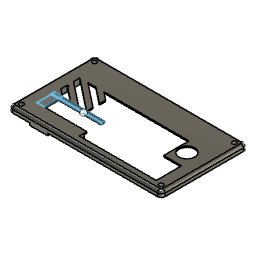
Untitled v9 (Autodesk Fusion 360 archive; units mm, degrees)
design "top"
Autodesk Fusion 360 part; units mm, degrees
sketch "Sketch1" plane through (0, 0, 0) normal (0, 0, 1) x (1, 0, 0)
  line L0 (0, 0) -> (119.41, 0)
  line L1 (119.41, 0) -> (119.41, 67.24)
  line L2 (119.41, 67.24) -> (0, 67.24)
  line L3 (0, 67.24) -> (0, 0)
  line L4 (0, 0) -> (5, 0)
  line L5 (5, 0) -> (5, 5)
  line L6 (5, 5) -> (0, 5)
  line L7 (0, 5) -> (0, 0)
  circle A0 centre (5, 5) radius 1.7
  line L8 (0, 67.24) -> (5, 67.24)
  line L9 (5, 67.24) -> (5, 62.24)
  line L10 (5, 62.24) -> (0, 62.24)
  line L11 (0, 62.24) -> (0, 67.24)
  circle A1 centre (5, 62.24) radius 1.7
  line L12 (119.41, 67.24) -> (114.41, 67.24)
  line L13 (114.41, 67.24) -> (114.41, 62.24)
  line L14 (114.41, 62.24) -> (119.41, 62.24)
  line L15 (119.41, 62.24) -> (119.41, 67.24)
  circle A2 centre (114.41, 62.24) radius 1.7
  line L16 (119.41, 0) -> (114.41, 0)
  line L17 (114.41, 0) -> (114.41, 5)
  line L18 (114.41, 5) -> (119.41, 5)
  line L19 (119.41, 5) -> (119.41, 0)
  circle A3 centre (114.41, 5) radius 1.7
  line L20 (0, 62.24) -> (10, 62.24)
  line L21 (0, 67.24) -> (10, 67.24)
  line L22 (10, 67.24) -> (10, 57.24)
  line L23 (10, 57.24) -> (0, 57.24)
  line L24 (0, 57.24) -> (0, 67.24)
  line L25 (0, 0) -> (10, 0)
  line L26 (10, 0) -> (10, 10)
  line L27 (10, 10) -> (0, 10)
  line L28 (0, 10) -> (0, 0)
  line L29 (119.41, 0) -> (109.41, 0)
  line L30 (109.41, 0) -> (109.41, 10)
  line L31 (109.41, 10) -> (119.41, 10)
  line L32 (119.41, 10) -> (119.41, 0)
  line L33 (10, 57.24) -> (109.41, 57.24)
  line L34 (109.41, 57.24) -> (109.41, 10)
  line L35 (109.41, 10) -> (10, 10)
  line L36 (10, 10) -> (10, 57.24)
  line L37 (109.41, 10) -> (109.41, 6.042)
  line L38 (109.41, 6.042) -> (49.127, 6.042)
  line L39 (49.127, 6.042) -> (49.127, 25.842)
  line L40 (49.127, 25.842) -> (109.41, 25.842)
  line L41 (109.41, 25.842) -> (109.41, 6.042)
  line L42 (109.41, 25.842) -> (95.41, 25.842)
  line L43 (95.41, 25.842) -> (35.127, 25.842)
  line L44 (35.127, 25.842) -> (35.127, 45.642)
  line L45 (35.127, 45.642) -> (95.41, 45.642)
  line L46 (95.41, 45.642) -> (95.41, 25.842)
  line L47 (35.127, 45.642) -> (10, 45.642)
  line L48 (10, 10) -> (49.127, 10)
  line L49 (49.127, 10) -> (49.127, 12)
  line L50 (49.127, 12) -> (10, 12)
  line L51 (10, 12) -> (10, 10)
  line L52 (10, 45.642) -> (11.5, 45.642)
  line L53 (11.5, 45.642) -> (11.5, 12)
  line L54 (11.5, 12) -> (10, 12)
  line L55 (10, 12) -> (10, 45.642)
  line L56 (35.127, 25.842) -> (10, 25.842)
  line L57 (22.5635, 45.642) -> (35.127, 35.742)
  line L58 (22.5635, 45.642) -> (10, 45.642)
  line L59 (35.127, 35.742) -> (35.127, 25.842)
  line L60 (16.2818, 45.642) -> (35.127, 30.792)
  line L61 (22.5635, 45.642) -> (35.127, 45.642)
  line L62 (28.8453, 45.642) -> (35.127, 40.692)
  line L63 (10, 45.642) -> (35.127, 25.842)
  line L64 (10, 45.642) -> (10, 25.842)
  line L65 (10, 45.642) -> (10, 33.62)
  line L66 (35.127, 35.742) -> (10, 35.742)
  line L67 (10, 45.642) -> (10, 35.742)
  line L68 (22.5635, 25.842) -> (35.127, 25.842)
  line L69 (28.8453, 25.842) -> (10, 40.692)
  line L70 (22.5635, 25.842) -> (10, 35.742)
  line L71 (10, 25.842) -> (22.5635, 25.842)
  line L72 (10, 35.742) -> (10, 25.842)
  line L73 (10, 30.792) -> (16.2817, 25.842)
  dimension "d1" = 119.41
  dimension "d2" = 67.24
  dimension "d3" = 5
  dimension "d4" = 5
  dimension "d5" = 3.4
  dimension "d6" = 5
  dimension "d7" = 5
  dimension "d8" = 3.4
  dimension "d9" = 5
  dimension "d10" = 5
  dimension "d11" = 3.4
  dimension "d12" = 5
  dimension "d13" = 5
  dimension "d14" = 3.4
  dimension "d15" = 10
  dimension "d16" = 10
  dimension "d17" = 10
  dimension "d18" = 10
  dimension "d19" = 10
  dimension "d20" = 10
  dimension "d21" = 3.958
  dimension "d22" = 60.283
  dimension "d23" = 19.8
  dimension "d24" = 14
  dimension "d25" = 60.283
  dimension "d26" = 19.8
  dimension "d27" = 2
  dimension "d28" = 1.5
  dimension "d29" = 90
  constraint horizontal L0
  constraint vertical L1
  constraint horizontal L2
  constraint vertical L3
  constraint coincident L0.start L3.end
  constraint horizontal L4
  constraint vertical L5
  constraint horizontal L6
  constraint vertical L7
  constraint coincident L5.end L6.start
  constraint horizontal L8
  constraint vertical L9
  constraint horizontal L10
  constraint vertical L11
  constraint coincident L9.end L10.start
  constraint horizontal L12
  constraint vertical L13
  constraint horizontal L14
  constraint vertical L15
  constraint coincident L13.end L14.start
  constraint horizontal L16
  constraint vertical L17
  constraint horizontal L18
  constraint vertical L19
  constraint coincident L17.end L18.start
  constraint perpendicular L11 L20
  constraint horizontal L21
  constraint vertical L22
  constraint horizontal L23
  constraint vertical L24
  constraint horizontal L25
  constraint vertical L26
  constraint horizontal L27
  constraint vertical L28
  constraint horizontal L29
  constraint vertical L30
  constraint horizontal L31
  constraint vertical L32
  constraint horizontal L33
  constraint vertical L34
  constraint horizontal L35
  constraint vertical L36
  constraint perpendicular L31 L37
  constraint horizontal L38
  constraint vertical L39
  constraint horizontal L40
  constraint vertical L41
  constraint perpendicular L41 L42
  constraint horizontal L43
  constraint vertical L44
  constraint horizontal L45
  constraint vertical L46
  constraint coincident L36 L47.end
  constraint perpendicular L36 L47
  constraint horizontal L48
  constraint vertical L49
  constraint horizontal L50
  constraint vertical L51
  constraint horizontal L52
  constraint vertical L53
  constraint horizontal L54
  constraint vertical L55
  constraint coincident L50 L53.end
  constraint coincident L36 L56.end
  constraint perpendicular L36 L56
  constraint midpoint L47 L57.start
  constraint midpoint L44 L57.end
  constraint midpoint L58 L60.start
  constraint midpoint L59 L60.end
  constraint midpoint L61 L62.start
  constraint coincident L44 L62.end
  constraint parallel L60 L62
  constraint midpoint L36 L65.end
  constraint coincident L65 L66.end
  constraint midpoint L56 L68.start
  constraint midpoint L68 L69.start
  constraint midpoint L67 L69.end
  constraint midpoint L72 L73.start
  constraint midpoint L71 L73.end
  measures "d1" distance of L0.start L0.end
  measures "d2" distance of L0.start L2.end
  measures "d3" distance of L0.start L4.end
  measures "d4" distance of L0.start L6.end
  measures "d5" diameter of A0
  measures "d6" distance of L2.end L8.end
  measures "d7" distance of L2.end L10.end
  measures "d8" diameter of A1
  measures "d9" distance of L1.end L12.end
  measures "d10" distance of L1.end L14.end
  measures "d11" diameter of A2
  measures "d12" distance of L0.end L16.end
  measures "d13" distance of L0.end L18.end
  measures "d14" diameter of A3
  measures "d15" distance of L2.end L21.end
  measures "d16" distance of L2.end L23.end
  measures "d17" distance of L0.start L25.end
  measures "d18" distance of L0.start L27.end
  measures "d19" distance of L0.end L29.end
  measures "d20" distance of L0.end L31.end
  measures "d21" distance of L30.end L37.end
  measures "d22" distance of L37.end L38.end
  measures "d23" distance of L37.end L40.end
  measures "d24" distance of L40.end L42.end
  measures "d25" distance of L42.end L43.end
  measures "d26" distance of L42.end L45.end
  measures "d27" distance of L26.end L50.end
  measures "d28" distance of L47.end L52.end
  measures "d29" angle of L65 L66
extrude "Extrude1" add sketch "Sketch1" against normal blind 4.5 contours L0 L3 L4 L5 L6 L7 A0 L25 L28 | L0 L3 L5 L6 A0 L25 L26 L27 L28 | L0 L26 L30 L35 L38 L39 L48 | L3 L23 L27 L36 L51 L55 L64 L65 L67 L72 | L0 L1 L17 L18 A3 L29 L30 L31 L32 L37 L41 | L3 L10 A1 L20 L22 L23 L24 | L0 L1 L16 L17 L18 L19 A3 L29 L32 | L2 L3 L8 L9 L10 L11 A1 L20 L21 L24 | L1 L2 L13 L14 A2 L22 L31 L33 L34 L41 | L2 L9 A1 L20 L21 L22 | L1 L2 L12 L13 L14 L15 A2
extrude "Extrude2" add sketch "Sketch1" against normal blind 1 contours L35 L36 L39 L48 L49 L50 L51 L54 | L33 L34 L36 L40 L42 L45 L46 L47 L52 L58 L61 | L36 L53 L55 L56 L64 L71 L72 L73 | L47 L52 L53 L58 L63 | L53 L56 L71 L73 | L36 L53 L55 L64 L65 L66 L67 L69 | L47 L53 L58 L60 L63 L66 | L44 L59 L60 L63 L66 | L53 L66 L69 | L53 L56 L66 L68 L69 L70 | L44 L47 L57 L61 L62
sketch "Sketch2" plane through (0, 0, 0) normal (0, 0, 1) x (1, 0, 0)
  line L0 (109.41, 25.8425) -> (95.4, 25.8425)
  line L1 (95.4, 25.8425) -> (95.4, 39.8525)
  line L2 (109.41, 39.8525) -> (109.41, 25.8425)
  line L3 (95.4, 39.8525) -> (96.4981, 39.8525)
  line L4 (108.3119, 39.8525) -> (109.41, 39.8525)
  circle A0 centre (102.405, 37.0367) radius 6.2407
  arc A1 (108.3977, 38.7785) -> (108.3119, 39.8525) centre (102.405, 38.8405) ccw
  arc A2 (96.4981, 39.8525) -> (96.4123, 38.7785) centre (102.405, 38.8405) ccw
  dimension "d34" = 14.01
  constraint horizontal L0
  constraint vertical L1
  constraint horizontal L3
  constraint vertical L2
  constraint collinear L3 L4
  constraint coincident L3.end A1
  constraint coincident A0 A1.start
  constraint coincident A0 A2.end
  constraint concentric A1 A2
  measures "d34" distance of L0.start L2.start
extrude "Extrude3" cut sketch "Sketch2" against normal blind 7 contours A0
sketch "Sketch3" plane through (0, 0, 0) normal (0, 0, 1) x (1, 0, 0)
  line L0 (10, 23.5) -> (35, 23.5)
  line L1 (10, 25.84) -> (49.1252, 25.84)
  line L2 (49.1252, 25.84) -> (49.1252, 23.5)
  line L3 (49.1252, 23.5) -> (10, 23.5)
  line L4 (10, 23.5) -> (10, 25.84)
  line L5 (10, 23.5) -> (49.1243, 23.5)
  line L6 (49.1243, 23.5) -> (49.1243, 23.0397)
  line L7 (49.1243, 23.0397) -> (10, 23.0397)
  line L8 (10, 23.0397) -> (10, 23.5)
  line L9 (10, 25.84) -> (16, 25.84)
  line L10 (16, 25.84) -> (16, 12)
  line L11 (16, 12) -> (10, 12)
  line L12 (10, 12) -> (10, 25.84)
  constraint horizontal L0
  constraint horizontal L1
  constraint vertical L2
  constraint horizontal L3
  constraint vertical L4
  constraint horizontal L5
  constraint vertical L6
  constraint horizontal L7
  constraint vertical L8
  constraint horizontal L9
  constraint vertical L10
  constraint horizontal L11
  constraint vertical L12
extrude "Extrude4" add sketch "Sketch3" against normal blind 1 contours L0 L1 L3 L4 L5 L9 L10 L12 | L0 L1 L2 L3 L5 L10
extrude "Extrude5" add sketch "Sketch3" against normal blind 1 contours L0 L3 L5 L7 L8 L10 L12 | L0 L3 L5 L6 L7 L10 | L7 L10 L11 L12
sketch "Sketch4" plane through (0, 0, 0) normal (0, -1, 0) x (1, 0, 0)
  line L0 (119.41, 0) -> (0, 0)
  line L1 (0, 0) -> (0, -4.5)
  line L2 (0, -4.5) -> (119.41, -4.5)
  line L3 (119.41, -4.5) -> (119.41, 0)
  line L4 (0, -4.5) -> (16.4, -4.5)
  line L5 (16.4, -4.5) -> (30.4, -4.5)
  line L6 (30.4, -4.5) -> (30.4, -6.214)
  line L7 (30.4, -6.214) -> (16.4, -6.214)
  line L8 (16.4, -6.214) -> (16.4, -4.5)
  dimension "d41" = 16.4
  dimension "d42" = 14
  dimension "d43" = 1.714
  constraint coincident L1.end L2.start
  constraint perpendicular L1 L4
  constraint horizontal L5
  constraint vertical L6
  constraint horizontal L7
  constraint vertical L8
  measures "d41" distance of L1.end L4.end
  measures "d42" distance of L4.end L5.end
  measures "d43" distance of L4.end L7.end
extrude "Extrude6" add sketch "Sketch4" against normal blind 5 contours L2 L5 L6 L7 L8
fillet "Fillet1" radius 3 4 edges at (119.41, 0, -2.25) (0, 67.24, -2.25) (0, 0, -2.25) (119.41, 67.24, -2.25)
fillet "Fillet2" radius 2 8 edges at (118.5313, 0.8787, 0) (119.41, 33.62, 0) (118.5313, 66.3613, 0) (59.705, 67.24, 0) (0.8787, 66.3613, 0) (0, 33.62, 0) (0.8787, 0.8787, 0) (59.705, 0, 0)
sketch "Sketch5" plane through (0, 0, -4.5) normal (0, 0, -1) x (1, 0, 0)
  arc A0 (116.41, -67.24) -> (119.41, -64.24) centre (116.41, -64.24) ccw
  line L0 (119.41, -64.24) -> (119.41, -3)
  arc A1 (119.41, -3) -> (116.41, 0) centre (116.41, -3) ccw
  line L1 (116.41, 0) -> (30.4, 0)
  line L2 (30.4, 0) -> (30.4, -5)
  line L3 (30.4, -5) -> (16.4, -5)
  line L4 (16.4, -5) -> (16.4, 0)
  line L5 (16.4, 0) -> (3, 0)
  arc A2 (3, 0) -> (0, -3) centre (3, -3) ccw
  line L6 (0, -3) -> (0, -64.24)
  arc A3 (0, -64.24) -> (3, -67.24) centre (3, -64.24) ccw
  line L7 (3, -67.24) -> (116.41, -67.24)
  circle A4 centre (114.41, -5) radius 1.7
  circle A5 centre (114.41, -62.24) radius 1.7
  circle A6 centre (5, -5) radius 1.7
  circle A7 centre (5, -62.24) radius 1.7
  line L8 (10, -45.642) -> (10, -35.742)
  line L9 (10, -35.742) -> (10, -25.842)
  line L10 (10, -25.842) -> (10, -10)
  line L11 (10, -10) -> (49.127, -10)
  line L12 (49.127, -10) -> (49.127, -6.042)
  line L13 (49.127, -6.042) -> (109.41, -6.042)
  line L14 (109.41, -6.042) -> (109.41, -57.24)
  line L15 (109.41, -57.24) -> (10, -57.24)
  line L16 (10, -57.24) -> (10, -45.642)
  line L17 (10, -67.24) -> (88.9145, -67.24) construction
  line L18 (88.9145, -67.24) -> (88.9145, -57.24) construction
  line L19 (88.9145, -57.24) -> (10, -57.24) construction
  line L20 (10, -57.24) -> (10, -67.24) construction
  dimension "d50" = 5
  text T0 "goonpad" font "Arial" height 5 align left top in box 78.9145 x 10 at (10, -67.24) x (1, 0) y (0, 1) spacing 1 kerned
  constraint coincident L7
  constraint coincident L15.end
extrude "Extrude7" cut sketch "Sketch5" against normal blind 0.2 text T0
